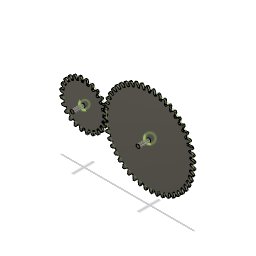
gears v4 (Autodesk Fusion 360 design; units mm, degrees)
description: Spur Gear; Diametrial Pitch: 2.000000; Num Teeth: 24; Pressure Angle: 20.000000; Backlash: 0.00 in
description: Spur Gear; Diametrial Pitch: 2.000000; Num Teeth: 48; Pressure Angle: 20.000000; Backlash: 0.00 in
Autodesk Fusion 360 part; units mm, degrees
(part 1 of 8)
sketch "Sketch1" plane through (0, 0, 0) normal (0, 0, 1) x (1, 0, 0) in component "Spur Gear (24 teeth)"
  circle A0 centre (0, 0) radius 137.1092
  circle A1 centre (0, 0) radius 12.7
extrude "Extrude1" add sketch "Sketch1" along normal blind 12.7 makes body 1 in component "Spur Gear (24 teeth)"
sketch "Sketch2" plane through (0, 0, 0) normal (0, 0, 1) x (1, 0, 0) in component "Spur Gear (24 teeth)"
  spline S0 degree 5 poles (142.7471, -11.4951) (142.8118, -11.5003) (142.9412, -11.509) (143.1354, -11.5173) (143.3946, -11.5189) (143.7188, -11.5082) (144.0433, -11.4883) (144.3678, -11.4628) (144.6924, -11.4343) (145.0169, -11.4038) (145.3415, -11.3711) (145.666, -11.3355) (145.9905, -11.2961) (146.3148, -11.2522) (146.6391, -11.2039) (146.9633, -11.1516) (147.2873, -11.0957) (147.6112, -11.037) (147.935, -10.9757) (148.2586, -10.9121) (148.5821, -10.846) (148.9053, -10.7774) (149.2285, -10.7062) (149.5514, -10.6322) (149.8741, -10.5555) (150.1966, -10.4762) (150.5189, -10.3945) (150.8411, -10.3105) (151.1629, -10.2242) (151.4846, -10.1358) (151.806, -10.0451) (152.1272, -9.9523) (152.4482, -9.8574) (152.7689, -9.7602) (153.0893, -9.661) (153.4095, -9.5596) (153.7295, -9.4562) (154.0491, -9.3508) (154.3685, -9.2434) (154.6877, -9.1341) (155.0065, -9.0228) (155.325, -8.9096) (155.6433, -8.7946) (155.9613, -8.6776) (156.279, -8.5588) (156.5963, -8.4382) (156.9134, -8.3157) (157.2301, -8.1914) (157.5466, -8.0654) (157.8627, -7.9376) (158.1785, -7.808) (158.494, -7.6767) (158.8091, -7.5437) (159.1239, -7.409) (159.4384, -7.2727) (159.7525, -7.1346) (160.0663, -6.9949) (160.3798, -6.8535) (160.6929, -6.7105) (161.0056, -6.5659) (161.318, -6.4196) (161.63, -6.2718) (161.9417, -6.1224) (162.253, -5.9714) (162.5639, -5.8189) (162.8745, -5.6648) (163.1846, -5.5091) (163.4944, -5.352) (163.8038, -5.1933) (164.1128, -5.0331) (164.4215, -4.8714) (164.6681, -4.7409) (164.8528, -4.6423) (164.9759, -4.5763) (165.0375, -4.5432) knots 0 0 0 0 0 0 0.01428571 0.02857143 0.04285714 0.05714286 0.07142857 0.08571429 0.1 0.11428571 0.12857143 0.14285714 0.15714286 0.17142857 0.18571429 0.2 0.21428571 0.22857143 0.24285714 0.25714286 0.27142857 0.28571429 0.3 0.31428571 0.32857143 0.34285714 0.35714286 0.37142857 0.38571429 0.4 0.41428571 0.42857143 0.44285714 0.45714286 0.47142857 0.48571429 0.5 0.51428571 0.52857143 0.54285714 0.55714286 0.57142857 0.58571429 0.6 0.61428571 0.62857143 0.64285714 0.65714286 0.67142857 0.68571429 0.7 0.71428571 0.72857143 0.74285714 0.75714286 0.77142857 0.78571429 0.8 0.81428571 0.82857143 0.84285714 0.85714286 0.87142857 0.88571429 0.9 0.91428571 0.92857143 0.94285714 0.95714286 0.97142857 0.98571429 1 1 1 1 1 1
  spline S1 degree 5 poles (142.7471, 11.4951) (142.8118, 11.5003) (142.9412, 11.509) (143.1354, 11.5173) (143.3946, 11.5189) (143.7188, 11.5082) (144.0433, 11.4883) (144.3678, 11.4628) (144.6924, 11.4343) (145.0169, 11.4038) (145.3415, 11.3711) (145.666, 11.3355) (145.9905, 11.2961) (146.3148, 11.2522) (146.6391, 11.2039) (146.9633, 11.1516) (147.2873, 11.0957) (147.6112, 11.037) (147.935, 10.9757) (148.2586, 10.9121) (148.5821, 10.846) (148.9053, 10.7774) (149.2285, 10.7062) (149.5514, 10.6322) (149.8741, 10.5555) (150.1966, 10.4762) (150.5189, 10.3945) (150.8411, 10.3105) (151.1629, 10.2242) (151.4846, 10.1358) (151.806, 10.0451) (152.1272, 9.9523) (152.4482, 9.8574) (152.7689, 9.7602) (153.0893, 9.661) (153.4095, 9.5596) (153.7295, 9.4562) (154.0491, 9.3508) (154.3685, 9.2434) (154.6877, 9.1341) (155.0065, 9.0228) (155.325, 8.9096) (155.6433, 8.7946) (155.9613, 8.6776) (156.279, 8.5588) (156.5963, 8.4382) (156.9134, 8.3157) (157.2301, 8.1914) (157.5466, 8.0654) (157.8627, 7.9376) (158.1785, 7.808) (158.494, 7.6767) (158.8091, 7.5437) (159.1239, 7.409) (159.4384, 7.2727) (159.7525, 7.1346) (160.0663, 6.9949) (160.3798, 6.8535) (160.6929, 6.7105) (161.0056, 6.5659) (161.318, 6.4196) (161.63, 6.2718) (161.9417, 6.1224) (162.253, 5.9714) (162.5639, 5.8189) (162.8745, 5.6648) (163.1846, 5.5091) (163.4944, 5.352) (163.8038, 5.1933) (164.1128, 5.0331) (164.4215, 4.8714) (164.6681, 4.7409) (164.8528, 4.6423) (164.9759, 4.5763) (165.0375, 4.5432) knots 0 0 0 0 0 0 0.01428571 0.02857143 0.04285714 0.05714286 0.07142857 0.08571429 0.1 0.11428571 0.12857143 0.14285714 0.15714286 0.17142857 0.18571429 0.2 0.21428571 0.22857143 0.24285714 0.25714286 0.27142857 0.28571429 0.3 0.31428571 0.32857143 0.34285714 0.35714286 0.37142857 0.38571429 0.4 0.41428571 0.42857143 0.44285714 0.45714286 0.47142857 0.48571429 0.5 0.51428571 0.52857143 0.54285714 0.55714286 0.57142857 0.58571429 0.6 0.61428571 0.62857143 0.64285714 0.65714286 0.67142857 0.68571429 0.7 0.71428571 0.72857143 0.74285714 0.75714286 0.77142857 0.78571429 0.8 0.81428571 0.82857143 0.84285714 0.85714286 0.87142857 0.88571429 0.9 0.91428571 0.92857143 0.94285714 0.95714286 0.97142857 0.98571429 1 1 1 1 1 1
  arc A0 (165.0375, -4.5432) -> (165.0375, 4.5432) centre (0, 0) ccw
  line L0 (136.6568, -11.0055) -> (142.7471, -11.4951)
  line L1 (136.6568, 11.0055) -> (142.7471, 11.4951)
  line L2 (136.6568, -11.0055) -> (136.6568, 11.0055)
  point P0 (144.318, -11.4661)
  point P1 (145.899, -11.3066)
  point P2 (147.486, -11.0593)
  point P3 (149.0774, -10.7392)
  point P4 (150.672, -10.3543)
  point P5 (152.2688, -9.9102)
  point P6 (153.8671, -9.4106)
  point P7 (155.466, -8.8584)
  point P8 (157.065, -8.256)
  point P9 (158.6633, -7.605)
  point P10 (160.2603, -6.9071)
  point P11 (161.8554, -6.1635)
  point P12 (163.448, -5.3752)
  point P13 (144.318, 11.4661)
  point P14 (145.899, 11.3066)
  point P15 (147.486, 11.0593)
  point P16 (149.0774, 10.7392)
  point P17 (150.672, 10.3543)
  point P18 (152.2688, 9.9102)
  point P19 (153.8671, 9.4106)
  point P20 (155.466, 8.8584)
  point P21 (157.065, 8.256)
  point P22 (158.6633, 7.605)
  point P23 (160.2603, 6.9071)
  point P24 (161.8554, 6.1635)
  point P25 (163.448, 5.3752)
extrude "Extrude2" add sketch "Sketch2" along normal blind 12.7 bodies 1 in component "Spur Gear (24 teeth)"
fillet "Fillet1" radius 1.5875 2 edges at (136.6667, -11.0062, 6.35) (136.6667, 11.0062, 6.35) on bodies 1 in component "Spur Gear (24 teeth)"
pattern_circular "C-Pattern1" count 24 over 360 about axis through (0, 0, 0) along (0, 0, 1) of "Extrude2", "Fillet1" in component "Spur Gear (24 teeth)"
sketch "Sketch3" plane through (0, 0, 0) normal (0, 0, 1) x (1, 0, 0) in component "Spur Gear (24 teeth)"
  circle A0 centre (0, 0) radius 152.4 construction
sketch "Sketch1 (2)" plane through (0, 0, 0) normal (0, 0, 1) x (1, 0, 0) in component "Spur Gear (48 teeth)"
  circle A0 centre (0, 0) radius 289.5092
  circle A1 centre (0, 0) radius 12.7
extrude "Extrude1'" add sketch "Sketch1 (2)" along normal blind 12.7 separate body makes body 2 in component "Spur Gear (48 teeth)"
sketch "Sketch2 (2)" plane through (0, 0, 0) normal (0, 0, 1) x (1, 0, 0) in component "Spur Gear (48 teeth)"
  spline S0 degree 5 poles (286.0935, -13.6367) (286.1846, -13.6371) (286.3669, -13.637) (286.6403, -13.6347) (287.0048, -13.6272) (287.4604, -13.6105) (287.916, -13.5865) (288.3716, -13.5554) (288.8272, -13.5177) (289.2826, -13.4738) (289.738, -13.4244) (290.1933, -13.3701) (290.6484, -13.3115) (291.1033, -13.2491) (291.558, -13.183) (292.0126, -13.1134) (292.4669, -13.0403) (292.921, -12.9637) (293.375, -12.8836) (293.8287, -12.8) (294.2822, -12.7131) (294.7355, -12.6231) (295.1886, -12.53) (295.6414, -12.434) (296.094, -12.3352) (296.5463, -12.2336) (296.9984, -12.1292) (297.4502, -12.0221) (297.9018, -11.9123) (298.3531, -11.7999) (298.8041, -11.6848) (299.2549, -11.5672) (299.7054, -11.4472) (300.1556, -11.3247) (300.6055, -11.1997) (301.0551, -11.0724) (301.5044, -10.9428) (301.9535, -10.8108) (302.4022, -10.6765) (302.8507, -10.54) (303.2988, -10.4012) (303.7466, -10.2603) (304.1942, -10.1171) (304.6414, -9.9718) (305.0883, -9.8244) (305.5349, -9.6749) (305.9811, -9.5233) (306.427, -9.3696) (306.8726, -9.2139) (307.3179, -9.0561) (307.7628, -8.8964) (308.2075, -8.7347) (308.6517, -8.571) (309.0956, -8.4053) (309.5392, -8.2377) (309.9825, -8.0683) (310.4253, -7.8969) (310.8679, -7.7236) (311.3101, -7.5485) (311.7519, -7.3715) (312.1934, -7.1927) (312.6345, -7.012) (313.0752, -6.8296) (313.5156, -6.6453) (313.9556, -6.4593) (314.3952, -6.2715) (314.8345, -6.0819) (315.2734, -5.8906) (315.7119, -5.6976) (316.15, -5.5028) (316.5878, -5.3063) (316.9377, -5.1478) (317.1999, -5.0281) (317.3747, -4.948) (317.4621, -4.9079) knots 0 0 0 0 0 0 0.01428571 0.02857143 0.04285714 0.05714286 0.07142857 0.08571429 0.1 0.11428571 0.12857143 0.14285714 0.15714286 0.17142857 0.18571429 0.2 0.21428571 0.22857143 0.24285714 0.25714286 0.27142857 0.28571429 0.3 0.31428571 0.32857143 0.34285714 0.35714286 0.37142857 0.38571429 0.4 0.41428571 0.42857143 0.44285714 0.45714286 0.47142857 0.48571429 0.5 0.51428571 0.52857143 0.54285714 0.55714286 0.57142857 0.58571429 0.6 0.61428571 0.62857143 0.64285714 0.65714286 0.67142857 0.68571429 0.7 0.71428571 0.72857143 0.74285714 0.75714286 0.77142857 0.78571429 0.8 0.81428571 0.82857143 0.84285714 0.85714286 0.87142857 0.88571429 0.9 0.91428571 0.92857143 0.94285714 0.95714286 0.97142857 0.98571429 1 1 1 1 1 1
  spline S1 degree 5 poles (286.0935, 13.6367) (286.1846, 13.6371) (286.3669, 13.637) (286.6403, 13.6347) (287.0048, 13.6272) (287.4604, 13.6105) (287.916, 13.5865) (288.3716, 13.5554) (288.8272, 13.5177) (289.2826, 13.4738) (289.738, 13.4244) (290.1933, 13.3701) (290.6484, 13.3115) (291.1033, 13.2491) (291.558, 13.183) (292.0126, 13.1134) (292.4669, 13.0403) (292.921, 12.9637) (293.375, 12.8836) (293.8287, 12.8) (294.2822, 12.7131) (294.7355, 12.6231) (295.1886, 12.53) (295.6414, 12.434) (296.094, 12.3352) (296.5463, 12.2336) (296.9984, 12.1292) (297.4502, 12.0221) (297.9018, 11.9123) (298.3531, 11.7999) (298.8041, 11.6848) (299.2549, 11.5672) (299.7054, 11.4472) (300.1556, 11.3247) (300.6055, 11.1997) (301.0551, 11.0724) (301.5044, 10.9428) (301.9535, 10.8108) (302.4022, 10.6765) (302.8507, 10.54) (303.2988, 10.4012) (303.7466, 10.2603) (304.1942, 10.1171) (304.6414, 9.9718) (305.0883, 9.8244) (305.5349, 9.6749) (305.9811, 9.5233) (306.427, 9.3696) (306.8726, 9.2139) (307.3179, 9.0561) (307.7628, 8.8964) (308.2075, 8.7347) (308.6517, 8.571) (309.0956, 8.4053) (309.5392, 8.2377) (309.9825, 8.0683) (310.4253, 7.8969) (310.8679, 7.7236) (311.3101, 7.5485) (311.7519, 7.3715) (312.1934, 7.1927) (312.6345, 7.012) (313.0752, 6.8296) (313.5156, 6.6453) (313.9556, 6.4593) (314.3952, 6.2715) (314.8345, 6.0819) (315.2734, 5.8906) (315.7119, 5.6976) (316.15, 5.5028) (316.5878, 5.3063) (316.9377, 5.1478) (317.1999, 5.0281) (317.3747, 4.948) (317.4621, 4.9079) knots 0 0 0 0 0 0 0.01428571 0.02857143 0.04285714 0.05714286 0.07142857 0.08571429 0.1 0.11428571 0.12857143 0.14285714 0.15714286 0.17142857 0.18571429 0.2 0.21428571 0.22857143 0.24285714 0.25714286 0.27142857 0.28571429 0.3 0.31428571 0.32857143 0.34285714 0.35714286 0.37142857 0.38571429 0.4 0.41428571 0.42857143 0.44285714 0.45714286 0.47142857 0.48571429 0.5 0.51428571 0.52857143 0.54285714 0.55714286 0.57142857 0.58571429 0.6 0.61428571 0.62857143 0.64285714 0.65714286 0.67142857 0.68571429 0.7 0.71428571 0.72857143 0.74285714 0.75714286 0.77142857 0.78571429 0.8 0.81428571 0.82857143 0.84285714 0.85714286 0.87142857 0.88571429 0.9 0.91428571 0.92857143 0.94285714 0.95714286 0.97142857 0.98571429 1 1 1 1 1 1
  arc A0 (317.4621, -4.9079) -> (317.4621, 4.9079) centre (0, 0) ccw
  line L0 (286.0935, 13.6367) -> (286.0935, -13.6367)
  point P0 (288.3198, -13.5576)
  point P1 (290.5533, -13.3231)
  point P2 (292.7909, -12.9851)
  point P3 (295.0315, -12.5619)
  point P4 (297.2742, -12.0635)
  point P5 (299.5185, -11.4967)
  point P6 (301.7636, -10.8663)
  point P7 (304.009, -10.1761)
  point P8 (306.2543, -9.4288)
  point P9 (308.4989, -8.627)
  point P10 (310.7424, -7.7724)
  point P11 (312.9844, -6.8668)
  point P12 (315.2245, -5.9115)
  point P13 (288.3198, 13.5576)
  point P14 (290.5533, 13.3231)
  point P15 (292.7909, 12.9851)
  point P16 (295.0315, 12.5619)
  point P17 (297.2742, 12.0635)
  point P18 (299.5185, 11.4967)
  point P19 (301.7636, 10.8663)
  point P20 (304.009, 10.1761)
  point P21 (306.2543, 9.4288)
  point P22 (308.4989, 8.627)
  point P23 (310.7424, 7.7724)
  point P24 (312.9844, 6.8668)
  point P25 (315.2245, 5.9115)
extrude "Extrude2'" add sketch "Sketch2 (2)" along normal blind 12.7 bodies 2 in component "Spur Gear (48 teeth)"
fillet "Fillet1'" radius 1.5875 2 edges at (289.1951, 13.4812, 6.35) (289.1951, -13.4812, 6.35) on bodies 2 in component "Spur Gear (48 teeth)"
pattern_circular "C-Pattern1'" count 48 over 360 about axis through (0, 0, 0) along (0, 0, 1) of "Extrude2'", "Fillet1'" in component "Spur Gear (48 teeth)"
sketch "Sketch3 (2)" plane through (0, 0, 0) normal (0, 0, 1) x (1, 0, 0) in component "Spur Gear (48 teeth)"
  circle A0 centre (0, 0) radius 304.8 construction
move_body "Move1" bodies 2 to x (0.965926, 0.258819, 0) y (-0.258819, 0.965926, 0) z (0, 0, 1) at (-2.3133, -4.6266, 0) in component "Spur Gear (48 teeth)"
sketch "Sketch1 (3)" plane through (0, 0, 12.7) normal (0, 0, 1) x (1, 0, 0)
  arc A0 (737.0909, 71.5504) -> (735.4834, 79.6322) centre (452.3696, 19.1166) ccw
  spline S0 degree 3 poles (736.4303, 81.4315) (736.2392, 81.3527) (736.0654, 81.2373) (735.7717, 80.9463) (735.6546, 80.7735) (735.5108, 80.4339) (735.4708, 80.2759) (735.4401, 79.9534) (735.4495, 79.7906) (735.4834, 79.6322) knots 0 0 0 0 0.062015 0.062015 0.12403 0.12403 0.172638 0.172638 0.221247 0.221247 0.221247 0.221247
  spline S1 degree 5 poles (736.4303, 81.4315) (736.4561, 81.4422) (736.5667, 81.4879) (736.762, 81.5693) (737.0416, 81.6873) (737.405, 81.8436) (737.826, 82.0284) (738.246, 82.2166) (738.6648, 82.4082) (739.0825, 82.6031) (739.4992, 82.8012) (739.9148, 83.0025) (740.3293, 83.2068) (740.7428, 83.414) (741.1554, 83.6239) (741.567, 83.8365) (741.9776, 84.0517) (742.3873, 84.2695) (742.796, 84.4899) (743.2037, 84.7128) (743.6105, 84.9382) (744.0164, 85.1661) (744.4214, 85.3963) (744.8254, 85.6289) (745.2286, 85.8638) (745.6308, 86.1009) (746.0322, 86.3402) (746.4327, 86.5818) (746.8323, 86.8255) (747.231, 87.0713) (747.6288, 87.3192) (748.0257, 87.5693) (748.4218, 87.8213) (748.8171, 88.0754) (749.2114, 88.3315) (749.6049, 88.5896) (749.9976, 88.8496) (750.3894, 89.1116) (750.7804, 89.3754) (751.1705, 89.6412) (751.5598, 89.9088) (751.9482, 90.1782) (752.3358, 90.4495) (752.7225, 90.7226) (753.1085, 90.9975) (753.4936, 91.2742) (753.8778, 91.5526) (754.2613, 91.8328) (754.6439, 92.1147) (755.0257, 92.3983) (755.4066, 92.6836) (755.7868, 92.9706) (756.1661, 93.2592) (756.5446, 93.5496) (756.9223, 93.8415) (757.2992, 94.1351) (757.6752, 94.4303) (758.0504, 94.7271) (758.4249, 95.0255) (758.7985, 95.3254) (759.1713, 95.6269) (759.5433, 95.93) (759.8402, 96.1737) (760.0625, 96.3572) (760.2106, 96.4798) (760.2846, 96.5412) knots 0.13851185 0.13851185 0.13851185 0.13851185 0.13851185 0.13851185 0.14285714 0.15714286 0.17142857 0.18571429 0.2 0.21428571 0.22857143 0.24285714 0.25714286 0.27142857 0.28571429 0.3 0.31428571 0.32857143 0.34285714 0.35714286 0.37142857 0.38571429 0.4 0.41428571 0.42857143 0.44285714 0.45714286 0.47142857 0.48571429 0.5 0.51428571 0.52857143 0.54285714 0.55714286 0.57142857 0.58571429 0.6 0.61428571 0.62857143 0.64285714 0.65714286 0.67142857 0.68571429 0.7 0.71428571 0.72857143 0.74285714 0.75714286 0.77142857 0.78571429 0.8 0.81428571 0.82857143 0.84285714 0.85714286 0.87142857 0.88571429 0.9 0.91428571 0.92857143 0.94285714 0.95714286 0.97142857 0.98571429 1 1 1 1 1 1
  arc A1 (760.2846, 96.5412) -> (757.7441, 106.0224) centre (452.3696, 19.1166) ccw
  spline S2 degree 5 poles (757.7441, 106.0224) (757.6493, 106.0386) (757.4598, 106.0708) (757.1755, 106.1185) (756.7965, 106.1811) (756.3228, 106.2575) (755.8492, 106.3323) (755.3757, 106.4052) (754.9022, 106.4764) (754.4289, 106.5458) (753.9556, 106.6134) (753.4824, 106.6793) (753.0094, 106.7433) (752.5364, 106.8054) (752.0636, 106.8658) (751.5909, 106.9242) (751.1183, 106.9808) (750.6458, 107.0355) (750.1735, 107.0884) (749.7014, 107.1393) (749.2294, 107.1883) (748.7576, 107.2353) (748.2859, 107.2804) (747.8144, 107.3236) (747.3431, 107.3647) (746.872, 107.4039) (746.401, 107.441) (745.9303, 107.4761) (745.4598, 107.5091) (744.9895, 107.54) (744.5195, 107.5689) (744.0496, 107.5956) (743.5801, 107.6202) (743.1107, 107.6427) (742.6417, 107.6629) (742.1729, 107.681) (741.7044, 107.6968) (741.2362, 107.7103) (740.7683, 107.7216) (740.3007, 107.7305) (739.8334, 107.7371) (739.3665, 107.7413) (738.9, 107.7432) (738.4337, 107.7426) (737.9679, 107.7395) (737.5025, 107.7338) (737.0375, 107.7257) (736.5729, 107.7148) (736.1087, 107.7013) (735.645, 107.6852) (735.1818, 107.6662) (734.7191, 107.6446) (734.2568, 107.6201) (733.7951, 107.5927) (733.334, 107.5624) (732.8734, 107.5289) (732.4135, 107.4922) (731.9543, 107.4521) (731.4958, 107.4086) (731.038, 107.3616) (730.581, 107.3112) (730.1881, 107.2648) (729.887, 107.2272) (729.6772, 107.2) (729.5585, 107.1843) (729.5308, 107.1806) knots -1 -1 -1 -1 -1 -1 -0.98571429 -0.97142857 -0.95714286 -0.94285714 -0.92857143 -0.91428571 -0.9 -0.88571429 -0.87142857 -0.85714286 -0.84285714 -0.82857143 -0.81428571 -0.8 -0.78571429 -0.77142857 -0.75714286 -0.74285714 -0.72857143 -0.71428571 -0.7 -0.68571429 -0.67142857 -0.65714286 -0.64285714 -0.62857143 -0.61428571 -0.6 -0.58571429 -0.57142857 -0.55714286 -0.54285714 -0.52857143 -0.51428571 -0.5 -0.48571429 -0.47142857 -0.45714286 -0.44285714 -0.42857143 -0.41428571 -0.4 -0.38571429 -0.37142857 -0.35714286 -0.34285714 -0.32857143 -0.31428571 -0.3 -0.28571429 -0.27142857 -0.25714286 -0.24285714 -0.22857143 -0.21428571 -0.2 -0.18571429 -0.17142857 -0.15714286 -0.14285714 -0.13851185 -0.13851185 -0.13851185 -0.13851185 -0.13851185 -0.13851185
  spline S3 degree 3 poles (727.8111, 108.2654) (727.8748, 108.0688) (727.9762, 107.8864) (728.2433, 107.5709) (728.4064, 107.4407) (728.7337, 107.2707) (728.8881, 107.2185) (729.2073, 107.1626) (729.3702, 107.1593) (729.5308, 107.1806) knots 0 0 0 0 0.062015 0.062015 0.12403 0.12403 0.172638 0.172638 0.221247 0.221247 0.221247 0.221247
  arc A2 (727.8111, 108.2654) -> (725.1624, 116.0682) centre (452.3696, 19.1166) ccw
  spline S4 degree 3 poles (725.8664, 117.9758) (725.6872, 117.8727) (725.5299, 117.7355) (725.2767, 117.4087) (725.1832, 117.2221) (725.085, 116.8667) (725.066, 116.7049) (725.0776, 116.381) (725.1082, 116.2209) (725.1624, 116.0682) knots 0 0 0 0 0.062015 0.062015 0.12403 0.12403 0.172638 0.172638 0.221247 0.221247 0.221247 0.221247
  spline S5 degree 5 poles (725.8664, 117.9758) (725.8906, 117.9897) (725.9943, 118.0495) (726.1773, 118.1556) (726.4391, 118.3092) (726.7789, 118.5115) (727.1723, 118.7497) (727.564, 118.9911) (727.9543, 119.2357) (728.343, 119.4835) (728.7302, 119.7343) (729.116, 119.9881) (729.5003, 120.2448) (729.8833, 120.5042) (730.2649, 120.7661) (730.6452, 121.0306) (731.0242, 121.2976) (731.402, 121.567) (731.7784, 121.8389) (732.1536, 122.1131) (732.5275, 122.3897) (732.9002, 122.6686) (733.2716, 122.9497) (733.6418, 123.2331) (734.0109, 123.5185) (734.3787, 123.8061) (734.7454, 124.0958) (735.1109, 124.3875) (735.4753, 124.6813) (735.8385, 124.9771) (736.2006, 125.2748) (736.5615, 125.5745) (736.9213, 125.8761) (737.28, 126.1796) (737.6375, 126.485) (737.994, 126.7922) (738.3494, 127.1013) (738.7036, 127.4121) (739.0568, 127.7248) (739.4089, 128.0392) (739.7599, 128.3553) (740.1098, 128.6731) (740.4587, 128.9927) (740.8065, 129.314) (741.1533, 129.6369) (741.499, 129.9614) (741.8436, 130.2876) (742.1872, 130.6155) (742.5297, 130.9449) (742.8712, 131.2759) (743.2117, 131.6085) (743.5511, 131.9427) (743.8895, 132.2784) (744.2269, 132.6156) (744.5632, 132.9543) (744.8986, 133.2946) (745.2329, 133.6364) (745.5661, 133.9796) (745.8984, 134.3243) (746.2297, 134.6704) (746.5599, 135.018) (746.8892, 135.3671) (747.1518, 135.6474) (747.3483, 135.8584) (747.4791, 135.9993) (747.5444, 136.0698) knots 0.13851185 0.13851185 0.13851185 0.13851185 0.13851185 0.13851185 0.14285714 0.15714286 0.17142857 0.18571429 0.2 0.21428571 0.22857143 0.24285714 0.25714286 0.27142857 0.28571429 0.3 0.31428571 0.32857143 0.34285714 0.35714286 0.37142857 0.38571429 0.4 0.41428571 0.42857143 0.44285714 0.45714286 0.47142857 0.48571429 0.5 0.51428571 0.52857143 0.54285714 0.55714286 0.57142857 0.58571429 0.6 0.61428571 0.62857143 0.64285714 0.65714286 0.67142857 0.68571429 0.7 0.71428571 0.72857143 0.74285714 0.75714286 0.77142857 0.78571429 0.8 0.81428571 0.82857143 0.84285714 0.85714286 0.87142857 0.88571429 0.9 0.91428571 0.92857143 0.94285714 0.95714286 0.97142857 0.98571429 1 1 1 1 1 1
  arc A3 (747.5444, 136.0698) -> (743.7881, 145.1383) centre (452.3696, 19.1166) ccw
  spline S6 degree 5 poles (743.7881, 145.1383) (743.692, 145.142) (743.4999, 145.1491) (743.2118, 145.1593) (742.8279, 145.1719) (742.3483, 145.1859) (741.869, 145.1982) (741.39, 145.2087) (740.9113, 145.2175) (740.4329, 145.2245) (739.9548, 145.2298) (739.4771, 145.2333) (738.9998, 145.235) (738.5227, 145.2349) (738.0461, 145.233) (737.5698, 145.2292) (737.0939, 145.2237) (736.6183, 145.2163) (736.1432, 145.207) (735.6684, 145.1958) (735.1941, 145.1828) (734.7201, 145.1679) (734.2466, 145.151) (733.7735, 145.1322) (733.3009, 145.1115) (732.8287, 145.0888) (732.3569, 145.0642) (731.8856, 145.0375) (731.4148, 145.0088) (730.9445, 144.9781) (730.4747, 144.9454) (730.0054, 144.9106) (729.5367, 144.8737) (729.0684, 144.8347) (728.6007, 144.7935) (728.1336, 144.7502) (727.667, 144.7047) (727.2011, 144.6571) (726.7357, 144.6071) (726.271, 144.555) (725.8068, 144.5005) (725.3434, 144.4438) (724.8806, 144.3847) (724.4184, 144.3232) (723.957, 144.2593) (723.4962, 144.193) (723.0363, 144.1242) (722.5771, 144.0528) (722.1187, 143.9789) (721.661, 143.9023) (721.2043, 143.8231) (720.7483, 143.7412) (720.2932, 143.6566) (719.839, 143.5692) (719.3858, 143.4789) (718.9335, 143.3856) (718.4824, 143.2892) (718.0323, 143.1895) (717.5834, 143.0865) (717.1357, 142.9802) (716.6891, 142.8705) (716.3057, 142.7732) (716.012, 142.6967) (715.8076, 142.6424) (715.692, 142.6113) (715.665, 142.6041) knots -1 -1 -1 -1 -1 -1 -0.98571429 -0.97142857 -0.95714286 -0.94285714 -0.92857143 -0.91428571 -0.9 -0.88571429 -0.87142857 -0.85714286 -0.84285714 -0.82857143 -0.81428571 -0.8 -0.78571429 -0.77142857 -0.75714286 -0.74285714 -0.72857143 -0.71428571 -0.7 -0.68571429 -0.67142857 -0.65714286 -0.64285714 -0.62857143 -0.61428571 -0.6 -0.58571429 -0.57142857 -0.55714286 -0.54285714 -0.52857143 -0.51428571 -0.5 -0.48571429 -0.47142857 -0.45714286 -0.44285714 -0.42857143 -0.41428571 -0.4 -0.38571429 -0.37142857 -0.35714286 -0.34285714 -0.32857143 -0.31428571 -0.3 -0.28571429 -0.27142857 -0.25714286 -0.24285714 -0.22857143 -0.21428571 -0.2 -0.18571429 -0.17142857 -0.15714286 -0.14285714 -0.13851185 -0.13851185 -0.13851185 -0.13851185 -0.13851185 -0.13851185
  spline S7 degree 3 poles (713.8184, 143.4551) (713.9072, 143.2684) (714.0316, 143.1009) (714.3376, 142.8229) (714.5163, 142.7151) (714.8629, 142.5893) (715.0228, 142.5577) (715.3466, 142.544) (715.5086, 142.5619) (715.665, 142.6041) knots 0 0 0 0 0.062015 0.062015 0.12403 0.12403 0.172638 0.172638 0.221247 0.221247 0.221247 0.221247
  arc A4 (713.8184, 143.4551) -> (710.1739, 150.8454) centre (452.3696, 19.1166) ccw
  spline S8 degree 3 poles (710.6229, 152.8285) (710.4587, 152.7029) (710.3206, 152.5464) (710.1123, 152.1893) (710.0439, 151.9922) (709.9929, 151.627) (709.9952, 151.464) (710.049, 151.1444) (710.1002, 150.9897) (710.1739, 150.8454) knots 0 0 0 0 0.062015 0.062015 0.12403 0.12403 0.172638 0.172638 0.221247 0.221247 0.221247 0.221247
  spline S9 degree 5 poles (710.6229, 152.8285) (710.645, 152.8455) (710.7401, 152.9183) (710.9076, 153.0474) (711.1471, 153.2338) (711.4577, 153.4788) (711.8166, 153.7663) (712.1735, 154.0568) (712.5285, 154.3502) (712.8815, 154.6466) (713.2327, 154.9458) (713.582, 155.2478) (713.9295, 155.5525) (714.2754, 155.8596) (714.6195, 156.1691) (714.9621, 156.481) (715.303, 156.7952) (715.6423, 157.1116) (715.9801, 157.4302) (716.3162, 157.7511) (716.6508, 158.0741) (716.9839, 158.3993) (717.3155, 158.7265) (717.6456, 159.0557) (717.9742, 159.3869) (718.3014, 159.7201) (718.6271, 160.0551) (718.9514, 160.3921) (719.2743, 160.7309) (719.5958, 161.0716) (719.9159, 161.414) (720.2347, 161.7583) (720.552, 162.1043) (720.868, 162.452) (721.1826, 162.8014) (721.496, 163.1525) (721.8079, 163.5053) (722.1186, 163.8598) (722.4279, 164.2158) (722.736, 164.5735) (723.0427, 164.9327) (723.3482, 165.2935) (723.6524, 165.6559) (723.9553, 166.0198) (724.2569, 166.3852) (724.5573, 166.7521) (724.8564, 167.1205) (725.1542, 167.4904) (725.4508, 167.8617) (725.7462, 168.2344) (726.0404, 168.6086) (726.3333, 168.9842) (726.6249, 169.3612) (726.9154, 169.7396) (727.2047, 170.1194) (727.4927, 170.5005) (727.7795, 170.883) (728.0652, 171.2668) (728.3496, 171.6519) (728.6329, 172.0383) (728.9149, 172.426) (729.1958, 172.8151) (729.4195, 173.1273) (729.5868, 173.3621) (729.6981, 173.5188) (729.7537, 173.5973) knots 0.13851185 0.13851185 0.13851185 0.13851185 0.13851185 0.13851185 0.14285714 0.15714286 0.17142857 0.18571429 0.2 0.21428571 0.22857143 0.24285714 0.25714286 0.27142857 0.28571429 0.3 0.31428571 0.32857143 0.34285714 0.35714286 0.37142857 0.38571429 0.4 0.41428571 0.42857143 0.44285714 0.45714286 0.47142857 0.48571429 0.5 0.51428571 0.52857143 0.54285714 0.55714286 0.57142857 0.58571429 0.6 0.61428571 0.62857143 0.64285714 0.65714286 0.67142857 0.68571429 0.7 0.71428571 0.72857143 0.74285714 0.75714286 0.77142857 0.78571429 0.8 0.81428571 0.82857143 0.84285714 0.85714286 0.87142857 0.88571429 0.9 0.91428571 0.92857143 0.94285714 0.95714286 0.97142857 0.98571429 1 1 1 1 1 1
  arc A5 (729.7537, 173.5973) -> (724.8458, 182.098) centre (452.3696, 19.1166) ccw
  spline S10 degree 5 poles (724.8458, 182.098) (724.7501, 182.089) (724.5587, 182.0711) (724.2717, 182.0436) (723.8894, 182.0059) (723.4121, 181.9572) (722.9353, 181.9068) (722.459, 181.8547) (721.9833, 181.8009) (721.5081, 181.7454) (721.0334, 181.6883) (720.5594, 181.6294) (720.0859, 181.5688) (719.6129, 181.5064) (719.1406, 181.4423) (718.6689, 181.3764) (718.1977, 181.3088) (717.7272, 181.2394) (717.2574, 181.1681) (716.7881, 181.0951) (716.3195, 181.0203) (715.8516, 180.9436) (715.3843, 180.8651) (714.9177, 180.7847) (714.4518, 180.7025) (713.9866, 180.6184) (713.5221, 180.5324) (713.0584, 180.4444) (712.5953, 180.3545) (712.1331, 180.2627) (711.6715, 180.1689) (711.2108, 180.0731) (710.7509, 179.9754) (710.2917, 179.8756) (709.8334, 179.7737) (709.3759, 179.6698) (708.9193, 179.5638) (708.4635, 179.4558) (708.0087, 179.3455) (707.5547, 179.2331) (707.1017, 179.1186) (706.6496, 179.0018) (706.1984, 178.8828) (705.7483, 178.7616) (705.2991, 178.638) (704.851, 178.5121) (704.4039, 178.3839) (703.958, 178.2532) (703.5131, 178.12) (703.0694, 177.9843) (702.6269, 177.8462) (702.1855, 177.7055) (701.7454, 177.5622) (701.3065, 177.4163) (700.8689, 177.2676) (700.4327, 177.1161) (699.998, 176.9616) (699.5648, 176.804) (699.1332, 176.6433) (698.7031, 176.4794) (698.2747, 176.3124) (697.9073, 176.1659) (697.6261, 176.0517) (697.4305, 175.9712) (697.3199, 175.9253) (697.2941, 175.9146) knots -1 -1 -1 -1 -1 -1 -0.98571429 -0.97142857 -0.95714286 -0.94285714 -0.92857143 -0.91428571 -0.9 -0.88571429 -0.87142857 -0.85714286 -0.84285714 -0.82857143 -0.81428571 -0.8 -0.78571429 -0.77142857 -0.75714286 -0.74285714 -0.72857143 -0.71428571 -0.7 -0.68571429 -0.67142857 -0.65714286 -0.64285714 -0.62857143 -0.61428571 -0.6 -0.58571429 -0.57142857 -0.55714286 -0.54285714 -0.52857143 -0.51428571 -0.5 -0.48571429 -0.47142857 -0.45714286 -0.44285714 -0.42857143 -0.41428571 -0.4 -0.38571429 -0.37142857 -0.35714286 -0.34285714 -0.32857143 -0.31428571 -0.3 -0.28571429 -0.27142857 -0.25714286 -0.24285714 -0.22857143 -0.21428571 -0.2 -0.18571429 -0.17142857 -0.15714286 -0.14285714 -0.13851185 -0.13851185 -0.13851185 -0.13851185 -0.13851185 -0.13851185
  spline S11 degree 3 poles (695.3523, 176.5173) (695.4646, 176.3438) (695.6098, 176.1939) (695.9495, 175.9582) (696.1408, 175.8747) (696.5008, 175.7953) (696.6635, 175.7848) (696.9863, 175.8134) (697.1445, 175.8523) (697.2941, 175.9146) knots 0 0 0 0 0.062015 0.062015 0.12403 0.12403 0.172638 0.172638 0.221247 0.221247 0.221247 0.221247
  arc A6 (695.3523, 176.5173) -> (690.7743, 183.3687) centre (452.3696, 19.1166) ccw
  spline S12 degree 3 poles (690.9606, 185.3934) (690.8142, 185.2474) (690.6977, 185.0743) (690.5378, 184.6931) (690.4958, 184.4886) (690.4928, 184.1199) (690.5164, 183.9586) (690.6114, 183.6488) (690.6824, 183.5021) (690.7743, 183.3687) knots 0 0 0 0 0.062015 0.062015 0.12403 0.12403 0.172638 0.172638 0.221247 0.221247 0.221247 0.221247
  spline S13 degree 5 poles (690.9606, 185.3934) (690.9803, 185.4131) (691.065, 185.4977) (691.2143, 185.6476) (691.4274, 185.8637) (691.7034, 186.1471) (692.0216, 186.479) (692.3376, 186.8136) (692.6512, 187.1508) (692.9626, 187.4907) (693.2717, 187.8333) (693.5786, 188.1783) (693.8834, 188.5257) (694.1862, 188.8753) (694.487, 189.2271) (694.7859, 189.581) (695.0829, 189.937) (695.378, 190.295) (695.6713, 190.655) (695.9627, 191.017) (696.2523, 191.381) (696.5401, 191.7468) (696.8261, 192.1145) (697.1104, 192.484) (697.393, 192.8553) (697.6739, 193.2283) (697.9531, 193.603) (698.2306, 193.9794) (698.5066, 194.3574) (698.7808, 194.7371) (699.0535, 195.1184) (699.3246, 195.5013) (699.594, 195.8858) (699.8619, 196.2718) (700.1283, 196.6593) (700.3931, 197.0483) (700.6563, 197.4388) (700.9181, 197.8308) (701.1783, 198.2242) (701.437, 198.619) (701.6943, 199.0152) (701.95, 199.4128) (702.2043, 199.8117) (702.4571, 200.2121) (702.7084, 200.6137) (702.9583, 201.0167) (703.2068, 201.421) (703.4538, 201.8266) (703.6995, 202.2334) (703.9436, 202.6415) (704.1864, 203.0509) (704.4278, 203.4615) (704.6678, 203.8734) (704.9064, 204.2864) (705.1436, 204.7007) (705.3794, 205.1162) (705.6139, 205.5328) (705.847, 205.9506) (706.0787, 206.3695) (706.3091, 206.7896) (706.5381, 207.2109) (706.7658, 207.6332) (706.9469, 207.972) (707.0821, 208.2266) (707.172, 208.3965) (707.2169, 208.4816) knots 0.13851185 0.13851185 0.13851185 0.13851185 0.13851185 0.13851185 0.14285714 0.15714286 0.17142857 0.18571429 0.2 0.21428571 0.22857143 0.24285714 0.25714286 0.27142857 0.28571429 0.3 0.31428571 0.32857143 0.34285714 0.35714286 0.37142857 0.38571429 0.4 0.41428571 0.42857143 0.44285714 0.45714286 0.47142857 0.48571429 0.5 0.51428571 0.52857143 0.54285714 0.55714286 0.57142857 0.58571429 0.6 0.61428571 0.62857143 0.64285714 0.65714286 0.67142857 0.68571429 0.7 0.71428571 0.72857143 0.74285714 0.75714286 0.77142857 0.78571429 0.8 0.81428571 0.82857143 0.84285714 0.85714286 0.87142857 0.88571429 0.9 0.91428571 0.92857143 0.94285714 0.95714286 0.97142857 0.98571429 1 1 1 1 1 1
  arc A7 (707.2169, 208.4816) -> (701.2414, 216.2689) centre (452.3696, 19.1166) ccw
  spline S14 degree 5 poles (701.2414, 216.2689) (701.1477, 216.2476) (700.9603, 216.2048) (700.6793, 216.1401) (700.3052, 216.0528) (699.8383, 215.9422) (699.3722, 215.83) (698.9068, 215.7162) (698.4421, 215.6008) (697.9782, 215.4838) (697.5151, 215.3651) (697.0528, 215.2449) (696.5912, 215.123) (696.1305, 214.9994) (695.6706, 214.8742) (695.2115, 214.7473) (694.7532, 214.6188) (694.2958, 214.4885) (693.8392, 214.3566) (693.3835, 214.2229) (692.9287, 214.0876) (692.4748, 213.9505) (692.0218, 213.8116) (691.5696, 213.6711) (691.1185, 213.5287) (690.6682, 213.3846) (690.2189, 213.2387) (689.7706, 213.0909) (689.3233, 212.9414) (688.877, 212.79) (688.4316, 212.6368) (687.9873, 212.4817) (687.5441, 212.3247) (687.1019, 212.1659) (686.6608, 212.0051) (686.2208, 211.8423) (685.7819, 211.6777) (685.3442, 211.511) (684.9076, 211.3423) (684.4722, 211.1717) (684.0379, 210.9989) (683.605, 210.8242) (683.1732, 210.6473) (682.7427, 210.4683) (682.3135, 210.2872) (681.8857, 210.1039) (681.4592, 209.9184) (681.0341, 209.7306) (680.6104, 209.5405) (680.1882, 209.3481) (679.7675, 209.1534) (679.3483, 208.9563) (678.9306, 208.7567) (678.5145, 208.5548) (678.1001, 208.3503) (677.6874, 208.1431) (677.2766, 207.9332) (676.8676, 207.7204) (676.4607, 207.5047) (676.0557, 207.2861) (675.6528, 207.0646) (675.3076, 206.8714) (675.0437, 206.7215) (674.8603, 206.6161) (674.7567, 206.5562) (674.7325, 206.5422) knots -1 -1 -1 -1 -1 -1 -0.98571429 -0.97142857 -0.95714286 -0.94285714 -0.92857143 -0.91428571 -0.9 -0.88571429 -0.87142857 -0.85714286 -0.84285714 -0.82857143 -0.81428571 -0.8 -0.78571429 -0.77142857 -0.75714286 -0.74285714 -0.72857143 -0.71428571 -0.7 -0.68571429 -0.67142857 -0.65714286 -0.64285714 -0.62857143 -0.61428571 -0.6 -0.58571429 -0.57142857 -0.55714286 -0.54285714 -0.52857143 -0.51428571 -0.5 -0.48571429 -0.47142857 -0.45714286 -0.44285714 -0.42857143 -0.41428571 -0.4 -0.38571429 -0.37142857 -0.35714286 -0.34285714 -0.32857143 -0.31428571 -0.3 -0.28571429 -0.27142857 -0.25714286 -0.24285714 -0.22857143 -0.21428571 -0.2 -0.18571429 -0.17142857 -0.15714286 -0.14285714 -0.13851185 -0.13851185 -0.13851185 -0.13851185 -0.13851185 -0.13851185
  spline S15 degree 3 poles (672.7286, 206.8863) (672.8627, 206.729) (673.0262, 206.5993) (673.3937, 206.41) (673.5942, 206.3521) (673.9616, 206.3204) (674.1242, 206.3312) (674.4405, 206.4017) (674.5923, 206.461) (674.7325, 206.5422) knots 0 0 0 0 0.062015 0.062015 0.12403 0.12403 0.172638 0.172638 0.221247 0.221247 0.221247 0.221247
  arc A8 (672.7286, 206.8863) -> (667.2955, 213.0816) centre (452.3696, 19.1166) ccw
  spline S16 degree 3 poles (667.2159, 215.1133) (667.0898, 214.9494) (666.997, 214.7626) (666.8881, 214.3637) (666.8732, 214.1556) (666.9184, 213.7896) (666.9628, 213.6328) (667.0975, 213.338) (667.187, 213.2018) (667.2955, 213.0816) knots 0 0 0 0 0.062015 0.062015 0.12403 0.12403 0.172638 0.172638 0.221247 0.221247 0.221247 0.221247
  spline S17 degree 5 poles (667.2159, 215.1133) (667.2329, 215.1354) (667.3059, 215.2303) (667.4343, 215.3984) (667.6174, 215.6404) (667.854, 215.9574) (668.1262, 216.3281) (668.3958, 216.701) (668.6627, 217.0763) (668.927, 217.454) (669.1888, 217.8339) (669.448, 218.216) (669.7049, 218.6002) (669.9595, 218.9864) (670.2118, 219.3745) (670.4619, 219.7644) (670.7099, 220.1561) (670.9558, 220.5495) (671.1995, 220.9447) (671.4412, 221.3417) (671.6808, 221.7403) (671.9184, 222.1406) (672.154, 222.5425) (672.3876, 222.9459) (672.6193, 223.3509) (672.8491, 223.7574) (673.077, 224.1653) (673.3031, 224.5747) (673.5273, 224.9856) (673.7497, 225.3978) (673.9702, 225.8114) (674.189, 226.2264) (674.406, 226.6428) (674.6212, 227.0605) (674.8347, 227.4794) (675.0464, 227.8997) (675.2565, 228.3212) (675.4648, 228.7439) (675.6715, 229.1679) (675.8765, 229.5931) (676.0798, 230.0195) (676.2814, 230.4471) (676.4815, 230.8758) (676.6799, 231.3057) (676.8766, 231.7368) (677.0718, 232.1689) (677.2654, 232.6022) (677.4573, 233.0365) (677.6478, 233.472) (677.8366, 233.9085) (678.0239, 234.346) (678.2096, 234.7846) (678.3937, 235.2243) (678.5764, 235.665) (678.7575, 236.1066) (678.9371, 236.5493) (679.1151, 236.993) (679.2917, 237.4376) (679.4668, 237.8833) (679.6404, 238.3298) (679.8125, 238.7773) (679.9831, 239.2258) (680.1184, 239.5853) (680.2192, 239.8554) (680.2861, 240.0356) (680.3195, 240.1258) knots 0.13851185 0.13851185 0.13851185 0.13851185 0.13851185 0.13851185 0.14285714 0.15714286 0.17142857 0.18571429 0.2 0.21428571 0.22857143 0.24285714 0.25714286 0.27142857 0.28571429 0.3 0.31428571 0.32857143 0.34285714 0.35714286 0.37142857 0.38571429 0.4 0.41428571 0.42857143 0.44285714 0.45714286 0.47142857 0.48571429 0.5 0.51428571 0.52857143 0.54285714 0.55714286 0.57142857 0.58571429 0.6 0.61428571 0.62857143 0.64285714 0.65714286 0.67142857 0.68571429 0.7 0.71428571 0.72857143 0.74285714 0.75714286 0.77142857 0.78571429 0.8 0.81428571 0.82857143 0.84285714 0.85714286 0.87142857 0.88571429 0.9 0.91428571 0.92857143 0.94285714 0.95714286 0.97142857 0.98571429 1 1 1 1 1 1
  arc A9 (680.3195, 240.1258) -> (673.3787, 247.0665) centre (452.3696, 19.1166) ccw
  spline S18 degree 5 poles (673.3787, 247.0665) (673.2886, 247.0332) (673.1084, 246.9662) (672.8383, 246.8654) (672.4788, 246.7301) (672.0303, 246.5595) (671.5828, 246.3874) (671.1362, 246.2138) (670.6906, 246.0388) (670.246, 245.8622) (669.8023, 245.6841) (669.3596, 245.5045) (668.9179, 245.3234) (668.4773, 245.1408) (668.0376, 244.9566) (667.599, 244.7709) (667.1614, 244.5836) (666.7249, 244.3948) (666.2895, 244.2044) (665.8551, 244.0124) (665.4219, 243.8188) (664.9897, 243.6237) (664.5587, 243.4269) (664.1288, 243.2285) (663.7001, 243.0285) (663.2725, 242.8268) (662.8461, 242.6235) (662.4209, 242.4185) (661.9969, 242.2119) (661.5741, 242.0035) (661.1526, 241.7935) (660.7324, 241.5817) (660.3134, 241.3682) (659.8958, 241.153) (659.4794, 240.936) (659.0644, 240.7173) (658.6508, 240.4967) (658.2385, 240.2743) (657.8277, 240.0501) (657.4183, 239.8241) (657.0103, 239.5962) (656.6038, 239.3664) (656.1989, 239.1347) (655.7954, 238.901) (655.3935, 238.6654) (654.9933, 238.4278) (654.5946, 238.1882) (654.1977, 237.9466) (653.8025, 237.7028) (653.409, 237.457) (653.0173, 237.209) (652.6274, 236.9588) (652.2394, 236.7065) (651.8532, 236.4519) (651.469, 236.1951) (651.0869, 235.9358) (650.7069, 235.6741) (650.3293, 235.4098) (649.954, 235.1428) (649.581, 234.8732) (649.2104, 234.601) (648.8934, 234.3644) (648.6514, 234.1813) (648.4833, 234.0529) (648.3884, 233.98) (648.3662, 233.9629) knots -1 -1 -1 -1 -1 -1 -0.98571429 -0.97142857 -0.95714286 -0.94285714 -0.92857143 -0.91428571 -0.9 -0.88571429 -0.87142857 -0.85714286 -0.84285714 -0.82857143 -0.81428571 -0.8 -0.78571429 -0.77142857 -0.75714286 -0.74285714 -0.72857143 -0.71428571 -0.7 -0.68571429 -0.67142857 -0.65714286 -0.64285714 -0.62857143 -0.61428571 -0.6 -0.58571429 -0.57142857 -0.55714286 -0.54285714 -0.52857143 -0.51428571 -0.5 -0.48571429 -0.47142857 -0.45714286 -0.44285714 -0.42857143 -0.41428571 -0.4 -0.38571429 -0.37142857 -0.35714286 -0.34285714 -0.32857143 -0.31428571 -0.3 -0.28571429 -0.27142857 -0.25714286 -0.24285714 -0.22857143 -0.21428571 -0.2 -0.18571429 -0.17142857 -0.15714286 -0.14285714 -0.13851185 -0.13851185 -0.13851185 -0.13851185 -0.13851185 -0.13851185
  spline S19 degree 3 poles (646.3345, 234.0425) (646.488, 233.9041) (646.667, 233.7969) (647.0561, 233.6571) (647.2625, 233.6259) (647.6308, 233.6424) (647.7907, 233.6744) (648.095, 233.7856) (648.2378, 233.8641) (648.3662, 233.9629) knots 0 0 0 0 0.062015 0.062015 0.12403 0.12403 0.172638 0.172638 0.221247 0.221247 0.221247 0.221247
  arc A10 (646.3345, 234.0425) -> (640.1393, 239.4756) centre (452.3696, 19.1166) ccw
  spline S20 degree 3 poles (639.7952, 241.4796) (639.6916, 241.3007) (639.6239, 241.1033) (639.568, 240.6936) (639.5804, 240.4853) (639.673, 240.1284) (639.7374, 239.9787) (639.9094, 239.7041) (640.016, 239.5807) (640.1393, 239.4756) knots 0 0 0 0 0.062015 0.062015 0.12403 0.12403 0.172638 0.172638 0.221247 0.221247 0.221247 0.221247
  spline S21 degree 5 poles (639.7952, 241.4796) (639.8092, 241.5037) (639.8691, 241.6074) (639.9745, 241.7908) (640.1244, 242.0546) (640.3176, 242.3998) (640.5391, 242.8028) (640.7577, 243.2077) (640.9734, 243.6147) (641.1861, 244.0236) (641.3961, 244.4344) (641.6032, 244.8471) (641.8077, 245.2616) (642.0097, 245.6777) (642.2092, 246.0953) (642.4063, 246.5146) (642.6011, 246.9353) (642.7935, 247.3575) (642.9836, 247.7811) (643.1713, 248.2062) (643.3569, 248.6327) (643.5402, 249.0606) (643.7213, 249.4897) (643.9003, 249.9202) (644.0771, 250.352) (644.2519, 250.785) (644.4246, 251.2192) (644.5953, 251.6546) (644.764, 252.0912) (644.9306, 252.5289) (645.0953, 252.9678) (645.258, 253.4078) (645.4188, 253.8489) (645.5777, 254.2911) (645.7347, 254.7344) (645.8898, 255.1787) (646.043, 255.624) (646.1944, 256.0703) (646.3439, 256.5177) (646.4916, 256.966) (646.6376, 257.4153) (646.7817, 257.8655) (646.924, 258.3167) (647.0646, 258.7688) (647.2034, 259.2218) (647.3405, 259.6757) (647.4759, 260.1306) (647.6095, 260.5863) (647.7415, 261.0428) (647.8717, 261.5002) (648.0003, 261.9585) (648.1272, 262.4176) (648.2524, 262.8775) (648.3759, 263.3383) (648.4978, 263.7998) (648.6181, 264.2622) (648.7367, 264.7253) (648.8538, 265.1892) (648.9692, 265.6538) (649.083, 266.1192) (649.1952, 266.5854) (649.3058, 267.0523) (649.393, 267.4264) (649.4577, 267.7073) (649.5006, 267.8947) (649.5219, 267.9885) knots 0.13851185 0.13851185 0.13851185 0.13851185 0.13851185 0.13851185 0.14285714 0.15714286 0.17142857 0.18571429 0.2 0.21428571 0.22857143 0.24285714 0.25714286 0.27142857 0.28571429 0.3 0.31428571 0.32857143 0.34285714 0.35714286 0.37142857 0.38571429 0.4 0.41428571 0.42857143 0.44285714 0.45714286 0.47142857 0.48571429 0.5 0.51428571 0.52857143 0.54285714 0.55714286 0.57142857 0.58571429 0.6 0.61428571 0.62857143 0.64285714 0.65714286 0.67142857 0.68571429 0.7 0.71428571 0.72857143 0.74285714 0.75714286 0.77142857 0.78571429 0.8 0.81428571 0.82857143 0.84285714 0.85714286 0.87142857 0.88571429 0.9 0.91428571 0.92857143 0.94285714 0.95714286 0.97142857 0.98571429 1 1 1 1 1 1
  arc A11 (649.5219, 267.9885) -> (641.7345, 273.9639) centre (452.3696, 19.1166) ccw
  spline S22 degree 5 poles (641.7345, 273.9639) (641.6495, 273.919) (641.4796, 273.8292) (641.225, 273.6939) (640.8862, 273.5129) (640.4638, 273.2852) (640.0426, 273.0561) (639.6225, 272.8258) (639.2036, 272.594) (638.7858, 272.3609) (638.3691, 272.1265) (637.9537, 271.8906) (637.5394, 271.6534) (637.1263, 271.4148) (636.7145, 271.1748) (636.3039, 270.9335) (635.8945, 270.6907) (635.4864, 270.4465) (635.0795, 270.2009) (634.6739, 269.9538) (634.2697, 269.7054) (633.8667, 269.4555) (633.465, 269.2041) (633.0647, 268.9513) (632.6657, 268.697) (632.2681, 268.4413) (631.8719, 268.1841) (631.4771, 267.9253) (631.0837, 267.6651) (630.6918, 267.4034) (630.3013, 267.1401) (629.9123, 266.8753) (629.5248, 266.609) (629.1388, 266.3411) (628.7543, 266.0716) (628.3714, 265.8005) (627.9901, 265.5279) (627.6104, 265.2536) (627.2323, 264.9777) (626.8559, 264.7001) (626.4812, 264.4209) (626.1082, 264.14) (625.737, 263.8574) (625.3675, 263.5731) (624.9998, 263.2871) (624.6339, 262.9993) (624.27, 262.7097) (623.908, 262.4183) (623.548, 262.1251) (623.19, 261.8299) (622.834, 261.5329) (622.4801, 261.234) (622.1283, 260.9332) (621.7786, 260.6304) (621.4312, 260.3256) (621.0862, 260.0187) (620.7437, 259.7096) (620.4038, 259.3983) (620.0665, 259.0846) (619.732, 258.7687) (619.4, 258.4504) (619.1166, 258.1745) (618.9006, 257.9613) (618.7507, 257.8121) (618.6661, 257.7274) (618.6464, 257.7076) knots -1 -1 -1 -1 -1 -1 -0.98571429 -0.97142857 -0.95714286 -0.94285714 -0.92857143 -0.91428571 -0.9 -0.88571429 -0.87142857 -0.85714286 -0.84285714 -0.82857143 -0.81428571 -0.8 -0.78571429 -0.77142857 -0.75714286 -0.74285714 -0.72857143 -0.71428571 -0.7 -0.68571429 -0.67142857 -0.65714286 -0.64285714 -0.62857143 -0.61428571 -0.6 -0.58571429 -0.57142857 -0.55714286 -0.54285714 -0.52857143 -0.51428571 -0.5 -0.48571429 -0.47142857 -0.45714286 -0.44285714 -0.42857143 -0.41428571 -0.4 -0.38571429 -0.37142857 -0.35714286 -0.34285714 -0.32857143 -0.31428571 -0.3 -0.28571429 -0.27142857 -0.25714286 -0.24285714 -0.22857143 -0.21428571 -0.2 -0.18571429 -0.17142857 -0.15714286 -0.14285714 -0.13851185 -0.13851185 -0.13851185 -0.13851185 -0.13851185 -0.13851185
  spline S23 degree 3 poles (616.6217, 257.5213) (616.7919, 257.4041) (616.9834, 257.3211) (617.3874, 257.2334) (617.596, 257.2294) (617.9591, 257.2938) (618.1134, 257.3464) (618.4007, 257.4963) (618.532, 257.5929) (618.6464, 257.7076) knots 0 0 0 0 0.062015 0.062015 0.12403 0.12403 0.172638 0.172638 0.221247 0.221247 0.221247 0.221247
  arc A12 (616.6217, 257.5213) -> (609.7703, 262.0993) centre (452.3696, 19.1166) ccw
  spline S24 degree 3 poles (609.1675, 264.0412) (609.0882, 263.8503) (609.0468, 263.6458) (609.0449, 263.2323) (609.0843, 263.0274) (609.2227, 262.6856) (609.3062, 262.5456) (609.5126, 262.2958) (609.6343, 262.1874) (609.7703, 262.0993) knots 0 0 0 0 0.062015 0.062015 0.12403 0.12403 0.172638 0.172638 0.221247 0.221247 0.221247 0.221247
  spline S25 degree 5 poles (609.1675, 264.0412) (609.1782, 264.067) (609.2241, 264.1775) (609.3047, 264.3731) (609.4189, 264.6543) (609.5654, 265.0217) (609.7324, 265.4502) (609.8963, 265.8802) (610.057, 266.3118) (610.2145, 266.745) (610.369, 267.1797) (610.5206, 267.6159) (610.6692, 268.0535) (610.8152, 268.4924) (610.9584, 268.9326) (611.0991, 269.3739) (611.2373, 269.8165) (611.373, 270.2601) (611.5061, 270.705) (611.6368, 271.1509) (611.7651, 271.598) (611.891, 272.0461) (612.0145, 272.4953) (612.1358, 272.9455) (612.2548, 273.3966) (612.3715, 273.8487) (612.4861, 274.3017) (612.5985, 274.7557) (612.7087, 275.2106) (612.8168, 275.6663) (612.9228, 276.123) (613.0267, 276.5804) (613.1285, 277.0388) (613.2283, 277.4979) (613.3261, 277.9578) (613.4219, 278.4186) (613.5157, 278.8801) (613.6075, 279.3424) (613.6974, 279.8054) (613.7853, 280.2692) (613.8713, 280.7336) (613.9555, 281.1988) (614.0377, 281.6647) (614.1181, 282.1313) (614.1966, 282.5986) (614.2733, 283.0665) (614.3481, 283.5351) (614.4211, 284.0044) (614.4923, 284.4743) (614.5618, 284.9448) (614.6294, 285.4159) (614.6953, 285.8876) (614.7594, 286.36) (614.8217, 286.8329) (614.8823, 287.3064) (614.9412, 287.7805) (614.9984, 288.2551) (615.0539, 288.7303) (615.1077, 289.2061) (615.1597, 289.6823) (615.2101, 290.1591) (615.2589, 290.6365) (615.2965, 291.0188) (615.324, 291.3057) (615.342, 291.4971) (615.3509, 291.5929) knots 0.13851185 0.13851185 0.13851185 0.13851185 0.13851185 0.13851185 0.14285714 0.15714286 0.17142857 0.18571429 0.2 0.21428571 0.22857143 0.24285714 0.25714286 0.27142857 0.28571429 0.3 0.31428571 0.32857143 0.34285714 0.35714286 0.37142857 0.38571429 0.4 0.41428571 0.42857143 0.44285714 0.45714286 0.47142857 0.48571429 0.5 0.51428571 0.52857143 0.54285714 0.55714286 0.57142857 0.58571429 0.6 0.61428571 0.62857143 0.64285714 0.65714286 0.67142857 0.68571429 0.7 0.71428571 0.72857143 0.74285714 0.75714286 0.77142857 0.78571429 0.8 0.81428571 0.82857143 0.84285714 0.85714286 0.87142857 0.88571429 0.9 0.91428571 0.92857143 0.94285714 0.95714286 0.97142857 0.98571429 1 1 1 1 1 1
  arc A13 (615.3509, 291.5929) -> (606.8503, 296.5007) centre (452.3696, 19.1166) ccw
  spline S26 degree 5 poles (606.8503, 296.5007) (606.7718, 296.4451) (606.615, 296.3339) (606.3803, 296.1666) (606.068, 295.9428) (605.679, 295.662) (605.2913, 295.3799) (604.9048, 295.0967) (604.5197, 294.8122) (604.1359, 294.5266) (603.7535, 294.2397) (603.3723, 293.9517) (602.9926, 293.6624) (602.6142, 293.372) (602.2372, 293.0803) (601.8616, 292.7874) (601.4874, 292.4932) (601.1147, 292.1979) (600.7433, 291.9013) (600.3735, 291.6034) (600.0051, 291.3043) (599.6382, 291.0039) (599.2727, 290.7023) (598.9088, 290.3994) (598.5465, 290.0952) (598.1857, 289.7898) (597.8264, 289.483) (597.4688, 289.175) (597.1127, 288.8656) (596.7583, 288.555) (596.4055, 288.243) (596.0544, 287.9297) (595.7049, 287.615) (595.3572, 287.299) (595.0112, 286.9817) (594.667, 286.663) (594.3245, 286.3429) (593.9839, 286.0214) (593.6451, 285.6985) (593.3081, 285.3742) (592.973, 285.0484) (592.6399, 284.7213) (592.3087, 284.3926) (591.9795, 284.0625) (591.6523, 283.731) (591.3271, 283.3979) (591.0041, 283.0633) (590.6832, 282.7271) (590.3646, 282.3894) (590.0481, 282.05) (589.734, 281.7091) (589.4221, 281.3666) (589.1125, 281.0224) (588.8054, 280.6766) (588.5008, 280.329) (588.1988, 279.9797) (587.8996, 279.6286) (587.6032, 279.2755) (587.3097, 278.9205) (587.0193, 278.5636) (586.7317, 278.2047) (586.4868, 277.8942) (586.3004, 277.6547) (586.1713, 277.4871) (586.0984, 277.3921) (586.0815, 277.3699) knots -1 -1 -1 -1 -1 -1 -0.98571429 -0.97142857 -0.95714286 -0.94285714 -0.92857143 -0.91428571 -0.9 -0.88571429 -0.87142857 -0.85714286 -0.84285714 -0.82857143 -0.81428571 -0.8 -0.78571429 -0.77142857 -0.75714286 -0.74285714 -0.72857143 -0.71428571 -0.7 -0.68571429 -0.67142857 -0.65714286 -0.64285714 -0.62857143 -0.61428571 -0.6 -0.58571429 -0.57142857 -0.55714286 -0.54285714 -0.52857143 -0.51428571 -0.5 -0.48571429 -0.47142857 -0.45714286 -0.44285714 -0.42857143 -0.41428571 -0.4 -0.38571429 -0.37142857 -0.35714286 -0.34285714 -0.32857143 -0.31428571 -0.3 -0.28571429 -0.27142857 -0.25714286 -0.24285714 -0.22857143 -0.21428571 -0.2 -0.18571429 -0.17142857 -0.15714286 -0.14285714 -0.13851185 -0.13851185 -0.13851185 -0.13851185 -0.13851185 -0.13851185
  spline S27 degree 3 poles (584.0984, 276.9209) (584.2825, 276.8269) (584.4832, 276.7697) (584.8952, 276.7354) (585.1026, 276.7587) (585.4541, 276.8699) (585.6002, 276.9422) (585.8654, 277.1284) (585.983, 277.2412) (586.0815, 277.3699) knots 0 0 0 0 0.062015 0.062015 0.12403 0.12403 0.172638 0.172638 0.221247 0.221247 0.221247 0.221247
  arc A14 (584.0984, 276.9209) -> (576.7081, 280.5655) centre (452.3696, 19.1166) ccw
  spline S28 degree 3 poles (575.857, 282.4121) (575.8032, 282.2125) (575.789, 282.0043) (575.841, 281.5941) (575.9069, 281.3961) (576.0887, 281.0753) (576.1897, 280.9474) (576.4269, 280.7266) (576.5617, 280.635) (576.7081, 280.5655) knots 0 0 0 0 0.062015 0.062015 0.12403 0.12403 0.172638 0.172638 0.221247 0.221247 0.221247 0.221247